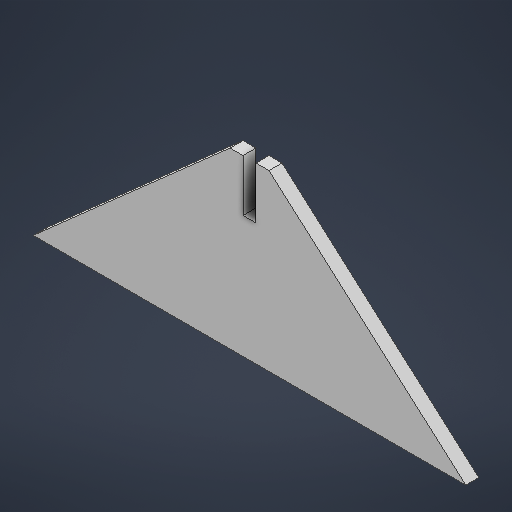
# Autodesk Inventor part: Base
Saved by Autodesk Inventor 2027 (Build 310192000, 192)
## iProperties
Created: 2026-05-24
Part Number: Base
Material: Generic
Document SubType Name: Modeling
Designer: alexy
Density: 1 g/cm^3
Appearance: Default
Author: alexy
Autodesk Inventor part; units mm, degrees
ref_plane "YZ Plane" through (0, 0, 0) normal (1, 0, 0) x (0, 1, 0)
ref_plane "XZ Plane" through (0, 0, 0) normal (0, 1, 0) x (-1, 0, 0)
ref_plane "XY Plane" through (0, 0, 0) normal (0, 0, 1) x (1, 0, 0)
sketch "Sketch1" plane through (0, 0, 0) normal (0, 0, 1) x (1, 0, 0)
  line L0 (0, 0) -> (0, 12)
  line L1 (0, 12) -> (0, 12)
  line L2 (0, 12) -> (0, 0)
  line L3 (0, 0) -> (3, 0)
  line L4 (3, 0) -> (3, 12)
  line L5 (3, 12) -> (6, 12)
  line L6 (6, 12) -> (51.5, -28.2336)
  line L7 (51.5, -28.2336) -> (-48.5, -28.2336)
  line L8 (0, 12) -> (-3, 12)
  line L9 (-3, 12) -> (-48.5, -28.2336)
  point P0 (1.5, 0)
  dimension "d0" = 3
  dimension "d1" = 12
  dimension "d2" = 3
  dimension "d3" = 3
  dimension "d4" = 100
  dimension "d5" = 50
  constraints: 20 end point, 4 perpendicular, 2 point on line, 1 coincident, 1 horizontal, 1 midpoint, 1 parallel, 1 vertical, 1 vertical alignment
  measures "d0" distance of L2.end L3.end
  measures "d1" distance of L3.end L4.end
  measures "d2" distance of L4.end L5.end
  measures "d3" distance of L1.end L8.end
  measures "d4" distance of L6.end L7.end
  measures "d5" horizontal distance of L7.end point (1.5, 0)
extrude "Extrusion1" add sketch "Sketch1" along normal blind 3
body "Solid1"
